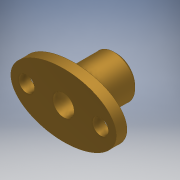
# Autodesk Inventor part: Glands
Saved by Autodesk Inventor 2017 (Build 210142000, 142)
## iProperties
Created: 2018-11-17
Part Number: Glands
Material: Brass, Soft Yellow
Document SubType Name: Modeling
Designer: Arman Grewal
Density: 8.47 g/cm^3
Appearance: Brass - Satin
Author: Arman Grewal
Autodesk Inventor part; units mm, degrees
ref_plane "YZ Plane" through (0, 0, 0) normal (1, 0, 0) x (0, 1, 0)
ref_plane "XZ Plane" through (0, 0, 0) normal (0, 1, 0) x (-1, 0, 0)
ref_plane "XY Plane" through (0, 0, 0) normal (0, 0, 1) x (1, 0, 0)
sketch "Sketch1" plane through (0, 0, 0) normal (0, 1, 0) x (-1, 0, 0)
  line L0 (0, 0) -> (-10, 0) construction
  line L1 (0, 0) -> (0, 6) construction
  ellipse E0 centre (0, 0) end of major axis (0, 6) minor radius 10 construction
  ellipse E1 centre (0, 0) end of major axis (0, -6) minor radius 10
  circle A0 centre (0, 0) radius 2
  circle A1 centre (7, 0) radius 1.5
  circle A2 centre (-7, 0) radius 1.5
  dimension "d7" = 6
  dimension "d0" = 10
  dimension "d1" = 6
  dimension "d2" = 4
  dimension "d3" = 3
  dimension "d4" = 3
  dimension "d5" = 7
  dimension "d6" = 7
  dimension "d8" = 7
  constraints: 4 end point, 3 centre point, 3 coincident, 2 vertical, 1 horizontal, 1 horizontal alignment, 1 point on line, 6 other
  measures "d0" distance of L0.start L0.end
  measures "d1" distance of L0.start L1.end
  measures "d2" diameter of A0
  measures "d3" diameter of A1
  measures "d4" diameter of A2
  measures "d5" distance of A1.centre L0.start
  measures "d6" distance of L0.start A2.centre
  measures "d8" distance from line of A1.centre L1
extrude "Extrusion1" add sketch "Sketch1" along normal blind 2
sketch "Sketch2" plane through (0, 2, 0) normal (0, 1, 0) x (1, 0, 0)
  circle A0 centre (0, 0) radius 4
  circle A1 centre (0, 0) radius 2
  dimension "d11" = 8
  dimension "d12" = 4
  constraints: 2 centre point, 2 coincident
  measures "d11" diameter of A0
  measures "d12" diameter of A1
extrude "Extrusion2" add sketch "Sketch2" along normal blind 8
chamfer "Chamfer1" distance 0.5 angle 45 2 edges at (-4, 10, 0) (-2, 10, 0)
body "Solid1"
